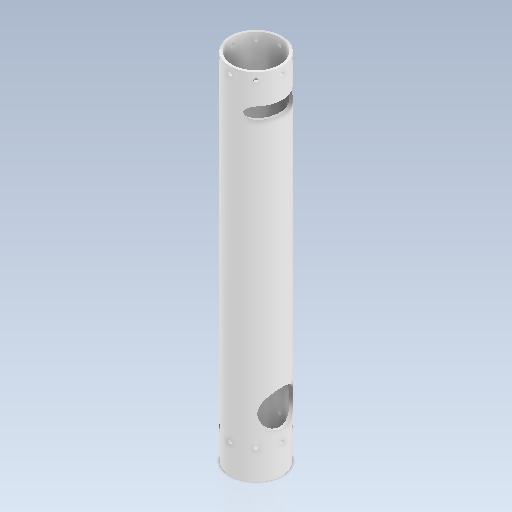
# Autodesk Inventor part: pvc30cm
Saved by Autodesk Inventor 2025.1 (Build 291241000, 241)
## iProperties
Created: 2024-11-07
Part Number: pvc30cm
Material: PVC-Piping
Document SubType Name: Modeling
Designer: ramad
Density: 1.4 g/cm^3
Appearance: Smooth - White
Author: ramad
Autodesk Inventor part; units mm, degrees
ref_plane "YZ Plane" through (0, 0, 0) normal (1, 0, 0) x (0, 1, 0)
ref_plane "XZ Plane" through (0, 0, 0) normal (0, 1, 0) x (-1, 0, 0)
ref_plane "XY Plane" through (0, 0, 0) normal (0, 0, 1) x (1, 0, 0)
sketch "Sketch1" plane through (0, 0, 0) normal (0, 1, 0) x (-1, 0, 0)
  circle A0 centre (0, 0) radius 20
  circle A1 centre (0, 0) radius 22
  dimension "d0" = 40
  dimension "d1" = 2
  constraints: 2 centre point, 1 coincident
  measures "d0" diameter of A0
  measures "d1" radial gap between concentric circles of A0 A1
extrude "Extrusion1" add sketch "Sketch1" along normal blind 300
sketch "Sketch2" plane through (0, 0, 0) normal (1, 0, 0) x (0, 1, 0)
  circle A0 centre (50, 0) radius 15
  line L0 (270, -15) -> (270, 15) construction
  line L1 (275, -15) -> (275, 15)
  line L2 (265, 15) -> (265, -15)
  arc A1 (265, -15) -> (275, -15) centre (270, -15) ccw
  arc A2 (275, 15) -> (265, 15) centre (270, 15) ccw
  line L3 (300, 20) -> (300, -20) projected
  circle A3 centre (25, 0) radius 1.5
  circle A4 centre (294, 0) radius 1.5
  point P0 (0, 0)
  point P1 (270, 0)
  dimension "d4" = 30
  dimension "d5" = 50
  dimension "d8" = 15
  dimension "d9" = 10
  dimension "d10" = 30
  dimension "d11" = 3
  dimension "d12" = 25
  dimension "d18" = 3
  dimension "d19" = 6
  constraints: 8 end point, 5 centre point, 4 point on circle, 4 tangent, 1 midpoint, 1 parallel, 1 vertical
  measures "d4" diameter of A0
  measures "d5" distance of point (0, 0) A0.centre
  measures "d8" distance of point (270, 0) L0.end
  measures "d9" diameter of A2
  measures "d10" distance from line of L3 point (270, 0)
  measures "d11" diameter of A3
  measures "d12" distance of point (0, 0) A3.centre
  measures "d18" diameter of A4
  measures "d19" distance from line of L3 A4.centre
extrude "Extrusion2" cut sketch "Sketch2" along normal up to surface contours A0 | A1 L2 A2 L1 round surface about axis through (0, 0, 0) along (0, 1, 0) radius 22 far side no
extrude "Extrusion3" cut sketch "Sketch2" along normal up to surface contours A3 round surface about axis through (0, 0, 0) along (0, 1, 0) radius 22 far side no
pattern_circular "Circular Pattern1" count 8 over 360 about axis through (0, 0, 0) along (0, 1, 0) of "Extrusion3"
extrude "Extrusion4" cut sketch "Sketch2" along normal up to surface contours A4 round surface about axis through (0, 0, 0) along (0, 1, 0) radius 22 far side no
pattern_circular "Circular Pattern2" count 8 over 360 about axis through (0, 0, 0) along (0, 1, 0) of "Extrusion4"
body "Solid1"
